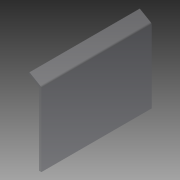
# Autodesk Inventor part: GE-13044
Saved by Autodesk Inventor 2013 (Build 170138000, 138)
## iProperties
Created: 2013-01-04
Part Number: GE-13044
Material: Polycarbonate, Clear
Document SubType Name: Modeling
Designer: Phillip
Density: 1 g/cm^3
Author: Phillip
Autodesk Inventor part; units mm, degrees
ref_plane "YZ Plane" through (0, 0, 0) normal (1, 0, 0) x (0, 1, 0)
ref_plane "XZ Plane" through (0, 0, 0) normal (0, 1, 0) x (-1, 0, 0)
ref_plane "XY Plane" through (0, 0, 0) normal (0, 0, 1) x (1, 0, 0)
sketch "Sketch1" plane through (0, 0, 0) normal (0, 0, 1) x (1, 0, 0)
  line L0 (0, 0) -> (6.35, 0)
  line L1 (6.35, 0) -> (6.35, 203.2)
  line L2 (6.35, 203.2) -> (-26.6456, 222.25)
  line L3 (-26.6456, 222.25) -> (-29.8206, 216.7507)
  line L4 (-29.8206, 216.7507) -> (-3.175, 201.3669)
  line L5 (0, 195.8677) -> (0, 0)
  arc A0 (6.35, 199.5338) -> (3.175, 205.0331) centre (0, 199.5338) ccw
  arc A1 (0, 195.8677) -> (-3.175, 201.3669) centre (-6.35, 195.8677) ccw
  dimension "d0" = 6.35
  dimension "d1" = 6.35
  dimension "d2" = 120
  dimension "d3" = 38.1
  dimension "d4" = 203.2
  dimension "d6" = 6.35
  constraints: 12 end point, 4 point on circle, 4 tangent, 3 perpendicular, 2 centre point, 2 point on line, 1 equal radius, 1 horizontal, 1 parallel
  measures "d0" distance of L0.start L0.end
  measures "d1" radius of A0
  measures "d2" angle of L5 L4
  measures "d3" distance from line of L1.end L3
  measures "d4" distance from line of L1.end L0
  measures "d6" distance of L2.end L3.end
extrude "Extrusion1" add sketch "Sketch1" against normal blind 304.8 contours L5 A1 L4 L3 L2 A0 L1 L0
body "Solid1"
